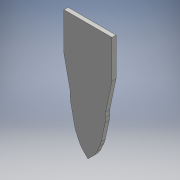
# Autodesk Inventor part: chasis
Saved by Autodesk Inventor 2016 (Build 200138000, 138)
## iProperties
Created: 2017-12-30
Part Number: chasis
Material: Genérico
Document SubType Name: Sheet Metal
Designer: David
Density: 1 g/cm^3
Sheet Metal Rule: Por defecto_mm
Appearance: Valor por defecto
Author: David
Autodesk Inventor part; units mm, degrees
ref_plane "YZ Plane" through (0, 0, 0) normal (1, 0, 0) x (0, 1, 0)
ref_plane "XZ Plane" through (0, 0, 0) normal (0, 1, 0) x (-1, 0, 0)
ref_plane "XY Plane" through (0, 0, 0) normal (0, 0, 1) x (1, 0, 0)
sketch "Boceto1" plane through (0, 0, 0) normal (0, 1, 0) x (-1, 0, 0)
  line L0 (0, 0) -> (-50, 0)
  line L1 (0, -84) -> (0, 0)
  line L2 (0, -84) -> (-14, -150)
  line L3 (-14, -150) -> (-14, -166)
  line L4 (-14, -166) -> (-25, -217)
  line L5 (-25, -217) -> (-37, -243)
  line L6 (-37, -243) -> (-53, -259)
  line L7 (-106, -84) -> (-106, 0)
  line L8 (-106, -84) -> (-92, -150)
  line L9 (-92, -150) -> (-92, -166)
  line L10 (-92, -166) -> (-81, -217)
  line L11 (-81, -217) -> (-69, -243)
  line L12 (-69, -243) -> (-53, -259)
  line L13 (0, 0) -> (-106, 0)
  constraints: 28 end point, 2 horizontal, 1 vertical
extrude "Extrusión1" add sketch "Boceto1" along normal blind 9
fillet "Empalme1" radius 50 1 edges at (92, 4.5, -166)
fillet "Empalme2" radius 50 1 edges at (14, 4.5, -166)
fillet "Empalme3" radius 50 4 edges at (25, 4.5, -217) (81, 4.5, -217) (69, 4.5, -243) (37, 4.5, -243)
equation "\"Radio_pliegue\" = Grosor"
equation "\"Anchura_desahogo_plegado\" = Grosor"
equation "\"Profundidad_desahogo_plegado\" = 0.5 * Grosor"
equation "\"Tamaño_destalonado\" = 4 * Grosor"
equation "\"Remanente_mínimo\" = 2 * Grosor"
equation "\"Radiodetransición\" = Radio_pliegue"
equation "\"Tamaño_de_radio_de_Jacobi\" = Radio_pliegue"
equation "\"TamañoSeparación\" = Grosor"
equation "\"Grosor\" = 0.5"
